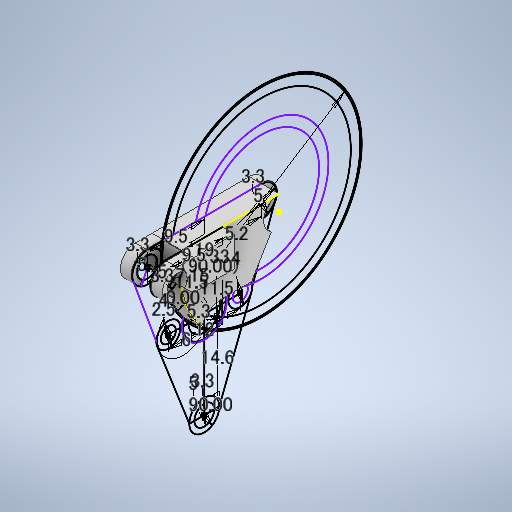
# Autodesk Inventor part: ikafly2c7
Saved by Autodesk Inventor 2025 (Build 290162000, 162)
## iProperties
Created: 2024-06-13
Part Number: ikafly2c7
Material: 一般
Document SubType Name: Modeling
Designer: Saigusa
Density: 1 g/cm^3
Appearance: 既定
Author: Saigusa
Autodesk Inventor part; units mm, degrees
ref_plane "YZ Plane" through (0, 0, 0) normal (1, 0, 0) x (0, 1, 0)
ref_plane "XZ Plane" through (0, 0, 0) normal (0, 1, 0) x (-1, 0, 0)
ref_plane "XY Plane" through (0, 0, 0) normal (0, 0, 1) x (1, 0, 0)
sketch "スケッチ1" plane through (0, 0, 0) normal (1, 0, 0) x (0, 1, 0)
  line L0 (0, 0) -> (0, 6)
  line L1 (0, 6) -> (0, -6)
  line L2 (0, 0) -> (11.5, 0)
  line L3 (11.5, 0) -> (11.5, 9.5)
  line L4 (11.5, 9.5) -> (11.5, -9.5)
  circle A0 centre (0, 6) radius 1.25
  circle A1 centre (0, -6) radius 1.25
  circle A2 centre (11.5, 9.5) radius 1.65
  circle A3 centre (11.5, -9.5) radius 1.65
  circle A4 centre (11.5, 9.5) radius 2.5
  circle A5 centre (11.5, -9.5) radius 2.5
  circle A6 centre (0, 0) radius 2.65
  line L5 (0, 0) -> (-14.6, 0)
  circle A7 centre (-14.6, 0) radius 1.65
  circle A8 centre (-14.6, 0) radius 2.5
  circle A9 centre (0, 6) radius 2
  circle A10 centre (0, -6) radius 2
  line L6 (0, 8) -> (10.6499, 11.851)
  line L7 (0, -8) -> (10.6499, -11.851)
  line L8 (-14.6, 0) -> (-14.6, -2.5)
  line L9 (-14.6, 0) -> (-12.1, 0) construction
  line L10 (-14.6, -2.5) -> (-14.6, 2.5)
  line L11 (-14.6, -2.5) -> (-0.7212, -7.8655)
  line L12 (-14.6, 2.5) -> (-0.7212, 7.8655)
  circle A11 centre (11.5, -9.5) radius 14.9164
  line L13 (11.5, -9.5) -> (0, 0)
  line L14 (11.5, -9.5) -> (0, -2.65)
  line L15 (14, 9.5) -> (14, 6.6979)
  circle A12 centre (11.5, -9.5) radius 16.7294
  circle A13 centre (11.5, -9.5) radius 2.6
  circle A14 centre (11.5, -9.5) radius 16.5
  line L16 (14, 6.6979) -> (14.1, -9.4839)
  line L17 (8.9, -9.5) -> (8.9, 0)
  line L18 (9, 9.5) -> (9, 0)
  line L19 (14.0414, 0) -> (11.5, 0)
  line L20 (0, 2.65) -> (2.65, 2.65)
  line L21 (2.65, 2.65) -> (2.65, 0)
  line L22 (2.65, 2.65) -> (2.65, 4.4258)
  circle A15 centre (0, 0) radius 3.575
  line L23 (0, 3.575) -> (14.0193, 3.575)
  line L24 (0, 3.575) -> (14.0193, 3.575) construction
  circle A16 centre (0, 0) radius 3.7299
  circle A17 centre (11.5, -9.5) radius 11.1866
  line L25 (0, -3.7299) -> (1.8129, -3.7299)
  line L26 (3.7299, 0) -> (3.7299, -4.8717)
  line L27 (3.7299, -3.7299) -> (1.8129, -3.7299)
  circle A18 centre (11.473, -9.4839) radius 9.6471
  line L28 (11.5, 9.5) -> (9.2001, 10.48)
  line L29 (11.5, 9.5) -> (9, 6.8095)
  point P0 (9.3522, -8.2206)
  point P1 (0, 2.65)
  point P2 (12.4812, 7.2006)
  point P3 (14, 6.8095)
  point P4 (0.3158, 2.6311)
  point P5 (9.2662, -8.1695)
  point P6 (1.3228, 3.4875)
  point P7 (2.6248, 2.65)
  point P8 (2.65, 2.6248)
  point P9 (1.3732, -3.4679)
  point P10 (3.1849, -4.5471)
  point P11 (11.5, 7.2294)
  point P12 (9, 7.0415)
  point P13 (9.9821, 10.1468)
  point P14 (11.5, 7.85)
  point P15 (9.2488, 7.0772)
  point P16 (10.3768, 8.2913)
  dimension "d9" = 5
  dimension "d32" = 7.15
  dimension "d0" = 6
  dimension "d1" = 12
  dimension "d2" = 11.5
  dimension "d3" = 9.5
  dimension "d4" = 19
  dimension "d5" = 2.5
  dimension "d6" = 3.3
  dimension "d7" = 3.3
  dimension "d8" = 5
  dimension "d10" = 5.3
  dimension "d11" = 14.6
  dimension "d12" = 3.3
  dimension "d13" = 5
  dimension "d14" = 4
  dimension "d15" = 4
  dimension "d16" = 90
  dimension "d21" = 5.2
  dimension "d22" = 33
  dimension "d33" = 0
  constraints: 60 end point, 19 point on circle, 19 point on line, 18 coincident, 14 centre point, 11 tangent, 8 perpendicular, 3 horizontal, 2 equal length, 1 parallel, 1 vertical, 1 vertical alignment, 15 other
  measures "d0" distance of L0.start L0.end
  measures "d1" distance of L0.end L1.end
  measures "d2" distance of L0.start L2.end
  measures "d3" distance of L2.end L3.end
  measures "d4" distance of L3.end L4.end
  measures "d5" diameter of A0
  measures "d6" diameter of A2
  measures "d7" diameter of A3
  measures "d8" diameter of A4
  measures "d10" diameter of A6
  measures "d11" distance of L5.start L5.end
  measures "d12" diameter of A7
  measures "d13" diameter of A8
  measures "d14" diameter of A9
  measures "d15" diameter of A10
  measures "d16" angle of L8 L9
  measures "d21" diameter of A13
  measures "d22" diameter of A14
  measures "d33" distance between parallel lines of L23 L24
extrude "押し出し3" add sketch "スケッチ1" along normal blind 3 contours L23 L22 L20 A16 A14 | A14 L22 L23 | L18 A11 L23 L22 A14 | A14 L3 A11 L18 | L23 A11 A16 L21 L22 | A14 L15 L16 A11 L3 | L18 L23 A11 | A11 L3 L23 L18 | L23 L18 A17 L2 A16 A11 | L2 A17 L26 | A11 L16 L23 L3 | L23 L3 A17 L18 | A17 L18 L2 | L2 L17 A18 L13 L26 A17 | L13 A18 L26 | L23 L16 A17 L3 | A17 L3 A18 L2 L18 | L2 A18 L17 | A18 L17 L13 | L13 L17 L14 L26 A18 | A17 L16 L19 A18 L3 | A18 L2 L4 A13 L13 L17 | L13 A13 L14 L17 | A18 L19 L3 | L3 L2 A18 | L19 A18 L16 A13 L4 | L19 L16 A18
extrude "押し出し4" add sketch "スケッチ1" against normal blind 2 contours L29 A4 A12 | A12 A4 A14 L29 | A14 L3 A11 L18 | A12 L3 A4 | A4 L29 A2 L3 A12 | A4 A12 L3 A2 L28 | A14 L15 L16 A11 L3 | L3 A12 A4 | A4 A12 L15 A14 | A11 L3 L23 L18 | A11 L16 L23 L3 | A4 L15 A12 | L23 L3 A17 L18 | L23 L16 A17 L3 | A17 L3 A18 L2 L18 | L2 A18 L17 | A17 L16 L19 A18 L3 | A18 L2 L4 A13 L13 L17 | L13 A13 L14 L17 | A18 L19 L3 | L3 L2 A18 | A13 L4 A5 L13 | L13 A5 L14 A13 | L14 A13 L17 | L19 A18 L16 A13 L4 | L19 L16 A18 | A13 L14 A5 L7 | L7 A5 L4 A13 | L13 A3 L14 A5 | A5 L4 A3 L13 | A5 L14 A3 L4
sketch "スケッチ3" plane through (3, 0, 0) normal (1, 0, 0) x (0, 0, -1)
  line L0 (0, 0) -> (0, 11.5)
  line L1 (0, 11.5) -> (-9.5, 11.5)
  circle A0 centre (-9.5, 11.5) radius 1.65
  circle A1 centre (-9.5, 11.5) radius 2.5
  line L2 (-10.1468, 9.9821) -> (-10.48, 9.2001) projected
  line L3 (-9.5, 11.5) -> (-10.48, 9.2001)
  line L4 (-9.5, 11.5) -> (-6.8095, 9)
  arc A2 (-6.8095, 14) -> (-3.4875, 1.3228) centre (9.5, 11.5) ccw projected
  line L5 (0, 9) -> (-6.8095, 9) projected
  line L6 (-6.8095, 9) -> (0, 9)
  line L7 (0, 9) -> (0, 14.0414)
  line L8 (9.4839, 14.1) -> (-6.6979, 14) projected
  line L9 (-9.5, 14) -> (-6.6979, 14) projected
  line L10 (-9.5, 14) -> (0, 14.0414)
  point P0 (-8.2913, 10.3768)
  dimension "d37" = 3.3
  dimension "d34" = 11.5
  dimension "d35" = 9.5
  dimension "d36" = 90
  dimension "d38" = 5
  constraints: 14 end point, 3 point on line, 2 coincident, 2 perpendicular, 1 centre point, 1 point on circle, 1 vertical, 2 other
  measures "d34" distance of L0.start L0.end
  measures "d35" distance of L0.end L1.end
  measures "d36" angle of L1 L0
  measures "d38" diameter of A1
extrude "押し出し6" add sketch "スケッチ3" along normal blind 2 contours L5 A2 L1 L0 | L1 A2 L9 L8 L7 | L4 A1 A2 | A1 L4 A0 L1 | L1 A0 L2 A1 | A1 L9 A2
extrude "押し出し7" cut sketch "スケッチ1" against normal blind 0.2 contours L29 A4 A12 | A12 A4 A14 L29 | A12 L3 A4 | A4 L29 A2 L3 A12 | A4 A12 L3 A2 L28 | L3 A12 A4 | A4 A12 L15 A14 | A4 L15 A12
extrude "押し出し8" cut sketch "スケッチ3" along normal blind 0.2 contours L4 A1 A2 | A1 L4 A0 L1 | L1 A0 L2 A1 | A1 L9 A2
